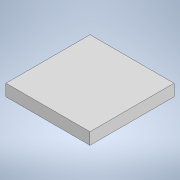
# Autodesk Inventor part: Part2
Saved by Autodesk Inventor 2021.1 (Build 251245000, 245)
## iProperties
Created: 2020-08-03
Part Number: Part2
Material: Generic
Document SubType Name: Modeling
Designer: adick
Density: 1 g/cm^3
Appearance: Default
Author: adick
Autodesk Inventor part; units mm, degrees
ref_plane "YZ Plane" through (0, 0, 0) normal (1, 0, 0) x (0, 1, 0)
ref_plane "XZ Plane" through (0, 0, 0) normal (0, 1, 0) x (-1, 0, 0)
ref_plane "XY Plane" through (0, 0, 0) normal (0, 0, 1) x (1, 0, 0)
sketch "Sketch1" plane through (0, 0, 0) normal (0, 1, 0) x (-1, 0, 0)
  line L0 (24, 24) -> (-24, 24)
  line L1 (-24, 24) -> (-24, -24)
  line L2 (-24, -24) -> (24, -24)
  line L3 (24, -24) -> (24, 24)
  line L4 (24, 24) -> (-24, -24) construction
  line L5 (-24, 24) -> (24, -24) construction
  line L6 (-25, 25) -> (25, 25)
  line L7 (25, 25) -> (25, -25)
  line L8 (25, -25) -> (-25, -25)
  line L9 (-25, -25) -> (-25, 25)
  line L10 (-25, 25) -> (25, -25) construction
  line L11 (25, 25) -> (-25, -25) construction
  point P0 (0, 0)
  constraints: 24 end point, 4 midpoint, 4 parallel, 2 horizontal, 2 perpendicular, 1 point on line
extrude "Extrusion1" add sketch "Sketch1" along normal blind 5
sketch "Sketch2" plane through (0, 5, 0) normal (0, 1, 0) x (1, 0, 0)
  line L0 (-25, -25) -> (25, -25) projected
  line L1 (25, 25) -> (-25, 25) projected
  line L2 (-25, -25) -> (25, -25)
  line L3 (25, -25) -> (25, 25)
  line L4 (25, 25) -> (-25, 25)
  line L5 (-25, 25) -> (-25, -25)
  point P0 (0, 0)
  constraints: 8 end point, 2 parallel, 1 horizontal, 1 perpendicular
extrude "Extrusion2" add sketch "Sketch2" along normal blind 2
sketch "Sketch3" plane through (0, 5, 0) normal (0, -1, 0) x (1, 0, 0)
  line L0 (24, -24) -> (24, 24) projected
  line L1 (24, 24) -> (-24, 24) projected
  line L2 (-24, -24) -> (24, -24) projected
  line L3 (-24, 24) -> (-24, -24) projected
  circle A0 centre (0, 0) radius 2.75
  line L4 (2.05, 0.585) -> (2.05, -0.585)
  line L5 (-2.05, -0.585) -> (-2.05, 0.585)
  line L6 (-0.585, 2.05) -> (0.585, 2.05)
  line L7 (0.585, -2.05) -> (-0.585, -2.05)
  line L8 (-2.05, 0.585) -> (-0.585, 0.585)
  line L9 (0.585, 0.585) -> (2.05, 0.585)
  line L10 (-0.585, -2.05) -> (-0.585, -0.585)
  line L11 (-0.585, 0.585) -> (-0.585, 2.05)
  line L12 (2.05, -0.585) -> (0.585, -0.585)
  line L13 (-0.585, -0.585) -> (-2.05, -0.585)
  line L14 (0.585, 2.05) -> (0.585, 0.585)
  line L15 (0.585, -0.585) -> (0.585, -2.05)
  constraints: 24 end point, 10 parallel, 4 perpendicular, 3 horizontal, 1 centre point, 1 coincident
extrude "Extrusion3" add sketch "Sketch3" along normal blind 3.9 contours A0
fillet "Fillet1" radius 0.3 4 edges at (0.585, 3.05, 0.585) (0.585, 3.05, -0.585) (-0.585, 3.05, 0.585) (-0.585, 3.05, -0.585)
fillet "Fillet2" radius 1.5 1 edges at (-2.75, 5, 0)
body "Solid1"
